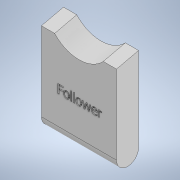
# Autodesk Inventor part: Follower
Saved by Autodesk Inventor 2021 (Build 250183000, 183)
## iProperties
Created: 2021-04-12
Part Number: Follower
Material: Generic
Document SubType Name: Modeling
Designer: Nabeel Azafer
Density: 1 g/cm^3
Appearance: Default
Author: Nabeel Azafer
Autodesk Inventor part; units mm, degrees
note: some values were not read from the file. Chosen so that the rebuilt part matches the saved one: direction of "Emboss1".
ref_plane "YZ Plane" through (0, 0, 0) normal (1, 0, 0) x (0, 1, 0)
ref_plane "XZ Plane" through (0, 0, 0) normal (0, 1, 0) x (-1, 0, 0)
sketch "Sketch1" plane through (0, 0, 0) normal (0, 0, 1) x (1, 0, 0)
  line L0 (0, 0) -> (17, 0)
  line L1 (17, 0) -> (17, 21.5)
  line L2 (17, 21.5) -> (0, 21.5)
  line L3 (0, 21.5) -> (0, 0)
  dimension "d0" = 17
  dimension "d1" = 21.5
  constraints: 8 end point, 2 parallel, 1 horizontal, 1 perpendicular
  measures "d0" distance of L0.start L0.end
  measures "d1" distance of L2.end L0.start
extrude "Extrusion1" add sketch "Sketch1" along normal blind 5
fillet "Fillet2" radius 2.5 2 edges at (8.5, 0, 5) (8.5, 0, 0)
ref_plane "Work Plane1" through (8.5, 21.5, 0) normal (-1, 0, 0) x (0, 0, 1)
sketch "Sketch5" plane through (8.5, 21.5, 0) normal (-1, 0, 0) x (0, 0, 1)
  line L0 (0, 0) -> (5, -1.1543)
  line L1 (5, -19) -> (5, 0) projected
  line L2 (0, 0) -> (5.1315, 0) construction
  point P0 (0, -21.5)
  dimension "d22" = 13
  constraints: 4 end point, 1 equal length, 1 horizontal, 1 point on line
  measures "d22" angle of L0 L2
sketch "Sketch6" plane through (0, 0, 0) normal (0, 0, -1) x (-1, 0, 0)
  line L0 (-14, 21.5) -> (-14, 24.5)
  line L1 (-14, 24.5) -> (-3, 24.5)
  line L2 (-3, 24.5) -> (-3, 21.5)
  line L3 (-17, 21.5) -> (0, 21.5) projected
  arc A0 (-14, 21.5) -> (-3, 21.5) centre (-8.5, 26.599) ccw
  point P0 (0, 0)
  dimension "d27" = 3
  dimension "d31" = 3
  dimension "d32" = 3
  dimension "d33" = 3
  dimension "d34" = 7.5
  constraints: 6 end point, 2 perpendicular, 2 point on circle, 1 centre point, 1 vertical
  measures "d27" distance of L0.start L0.end
  measures "d31" distance from line of L3.end L2
  measures "d32" distance between parallel lines of L3 L1
  measures "d33" distance of L1.end L2.end
  measures "d34" radius of A0
sweep "Sweep1" cut profiles "Sketch6" path "Sketch5" path curves L0
sketch "Sketch8" plane through (17, 21.5, 5) normal (1, 0, 0) x (0, 0, -1)
  line L0 (5, 0) -> (0, 0) projected
  line L1 (5, 0) -> (0, -1.1543) projected
  line L2 (5, 0) -> (0, -1.1543)
  line L3 (0, -19) -> (0, 0) projected
  line L4 (0, -1.1543) -> (0, 0)
  line L5 (0, 0) -> (5, 0)
  point P0 (5, -21.5)
  constraints: 6 end point, 2 collinear, 1 perpendicular
extrude "Extrusion6" cut sketch "Sketch8" against normal blind 17
sketch "Sketch9" plane through (0, 0, 5) normal (0, 0, 1) x (1, 0, 0)
  line L0 (3.5412, 10.9902) -> (19.7264, 10.9902) construction
  line L1 (19.7264, 10.9902) -> (19.7264, 4.3416) construction
  line L2 (19.7264, 4.3416) -> (3.5412, 4.3416) construction
  line L3 (3.5412, 4.3416) -> (3.5412, 10.9902) construction
  line L4 (4.9399, 10.6645) -> (4.0096, 10.6645)
  line L5 (4.0096, 10.6645) -> (4.0096, 10.1004)
  line L6 (4.0096, 10.1004) -> (4.901, 10.1004)
  line L7 (4.901, 10.1004) -> (4.901, 9.8638)
  line L8 (4.901, 9.8638) -> (4.0096, 9.8638)
  line L9 (4.0096, 9.8638) -> (4.0096, 8.9011)
  line L10 (4.0096, 8.9011) -> (3.7438, 8.9011)
  line L11 (3.7438, 8.9011) -> (3.7438, 10.9011)
  line L12 (3.7438, 10.9011) -> (4.9399, 10.9011)
  line L13 (4.9399, 10.9011) -> (4.9399, 10.6645)
  spline S0 degree 2 poles (6.3921, 9.6515) (6.3921, 9.2722) (6.0275, 8.859) (5.7228, 8.859) knots 0 0 0 1 2 2 2
  spline S1 degree 2 poles (5.7228, 8.859) (5.41, 8.859) (5.0518, 9.2852) (5.0518, 9.6515) knots 0 0 0 1 2 2 2
  spline S2 degree 2 poles (5.0518, 9.6515) (5.0518, 10.0275) (5.4213, 10.444) (5.7228, 10.444) knots 0 0 0 1 2 2 2
  spline S3 degree 2 poles (5.7228, 10.444) (6.0275, 10.444) (6.3921, 10.0291) (6.3921, 9.6515) knots 0 0 0 1 2 2 2
  spline S4 degree 2 poles (6.1312, 9.6515) (6.1312, 9.9432) (5.9189, 10.2269) (5.7228, 10.2269) knots 0 0 0 1 2 2 2
  spline S5 degree 2 poles (5.7228, 10.2269) (5.5266, 10.2269) (5.3127, 9.9432) (5.3127, 9.6515) knots 0 0 0 1 2 2 2
  spline S6 degree 2 poles (5.3127, 9.6515) (5.3127, 9.3679) (5.5266, 9.0761) (5.7228, 9.0761) knots 0 0 0 1 2 2 2
  spline S7 degree 2 poles (5.7228, 9.0761) (5.9172, 9.0761) (6.1312, 9.363) (6.1312, 9.6515) knots 0 0 0 1 2 2 2
  line L14 (6.9091, 8.9011) -> (6.6563, 8.9011)
  line L15 (6.6563, 8.9011) -> (6.6563, 10.9902)
  line L16 (6.6563, 10.9902) -> (6.9091, 10.9902)
  line L17 (6.9091, 10.9902) -> (6.9091, 8.9011)
  line L18 (7.538, 8.9011) -> (7.2852, 8.9011)
  line L19 (7.2852, 8.9011) -> (7.2852, 10.9902)
  line L20 (7.2852, 10.9902) -> (7.538, 10.9902)
  line L21 (7.538, 10.9902) -> (7.538, 8.9011)
  spline S8 degree 2 poles (9.1425, 9.6515) (9.1425, 9.2722) (8.7779, 8.859) (8.4732, 8.859) knots 0 0 0 1 2 2 2
  spline S9 degree 2 poles (8.4732, 8.859) (8.1604, 8.859) (7.8022, 9.2852) (7.8022, 9.6515) knots 0 0 0 1 2 2 2
  spline S10 degree 2 poles (7.8022, 9.6515) (7.8022, 10.0275) (8.1717, 10.444) (8.4732, 10.444) knots 0 0 0 1 2 2 2
  spline S11 degree 2 poles (8.4732, 10.444) (8.7779, 10.444) (9.1425, 10.0291) (9.1425, 9.6515) knots 0 0 0 1 2 2 2
  spline S12 degree 2 poles (8.8816, 9.6515) (8.8816, 9.9432) (8.6693, 10.2269) (8.4732, 10.2269) knots 0 0 0 1 2 2 2
  spline S13 degree 2 poles (8.4732, 10.2269) (8.2771, 10.2269) (8.0631, 9.9432) (8.0631, 9.6515) knots 0 0 0 1 2 2 2
  spline S14 degree 2 poles (8.0631, 9.6515) (8.0631, 9.3679) (8.2771, 9.0761) (8.4732, 9.0761) knots 0 0 0 1 2 2 2
  spline S15 degree 2 poles (8.4732, 9.0761) (8.6677, 9.0761) (8.8816, 9.363) (8.8816, 9.6515) knots 0 0 0 1 2 2 2
  line L22 (11.2203, 10.4019) -> (10.8395, 8.9011)
  line L23 (10.8395, 8.9011) -> (10.6061, 8.9011)
  line L24 (10.6061, 8.9011) -> (10.2398, 10.0583)
  line L25 (10.2398, 10.0583) -> (9.8751, 8.9011)
  line L26 (9.8751, 8.9011) -> (9.6433, 8.9011)
  line L27 (9.6433, 8.9011) -> (9.2592, 10.4019)
  line L28 (9.2592, 10.4019) -> (9.5218, 10.4019)
  line L29 (9.5218, 10.4019) -> (9.7876, 9.2398)
  line L30 (9.7876, 9.2398) -> (10.1425, 10.4019)
  line L31 (10.1425, 10.4019) -> (10.3516, 10.4019)
  line L32 (10.3516, 10.4019) -> (10.7163, 9.2398)
  line L33 (10.7163, 9.2398) -> (10.9659, 10.4019)
  line L34 (10.9659, 10.4019) -> (11.2203, 10.4019)
  spline S16 degree 2 poles (12.0939, 8.8671) (11.7341, 8.8671) (11.3386, 9.2706) (11.3386, 9.6434) knots 0 0 0 1 2 2 2
  spline S17 degree 2 poles (11.3386, 9.6434) (11.3386, 10.0097) (11.7228, 10.444) (12.0323, 10.444) knots 0 0 0 1 2 2 2
  spline S18 degree 2 poles (12.0323, 10.444) (12.1717, 10.444) (12.3873, 10.363) (12.4667, 10.2771) knots 0 0 0 1 2 2 2
  spline S19 degree 2 poles (12.4667, 10.2771) (12.5477, 10.1912) (12.6336, 9.9432) (12.6336, 9.7633) knots 0 0 0 1 2 2 2
  line L35 (12.6336, 9.7633) -> (12.6336, 9.6256)
  line L36 (12.6336, 9.6256) -> (11.5947, 9.6256)
  spline S20 degree 2 poles (11.5947, 9.6256) (11.5947, 9.3646) (11.8573, 9.0875) (12.0907, 9.0875) knots 0 0 0 1 2 2 2
  spline S21 degree 2 poles (12.0907, 9.0875) (12.1733, 9.0875) (12.3338, 9.1248) (12.3986, 9.1539) knots 0 0 0 1 2 2 2
  spline S22 degree 2 poles (12.3986, 9.1539) (12.4667, 9.1863) (12.5607, 9.2431) (12.5915, 9.269) knots 0 0 0 1 2 2 2
  line L37 (12.5915, 9.269) -> (12.6061, 9.269)
  line L38 (12.6061, 9.269) -> (12.6061, 8.9935)
  spline S23 degree 2 poles (12.6061, 8.9935) (12.5623, 8.9756) (12.4294, 8.9238) (12.3775, 8.9092) knots 0 0 0 1 2 2 2
  spline S24 degree 2 poles (12.3775, 8.9092) (12.3046, 8.8881) (12.1847, 8.8671) (12.0939, 8.8671) knots 0 0 0 1 2 2 2
  spline S25 degree 2 poles (12.3873, 9.8184) (12.384, 9.9205) (12.3419, 10.0696) (12.3014, 10.1199) knots 0 0 0 1 2 2 2
  spline S26 degree 2 poles (12.3014, 10.1199) (12.2576, 10.1766) (12.1198, 10.2366) (12.0177, 10.2366) knots 0 0 0 1 2 2 2
  spline S27 degree 2 poles (12.0177, 10.2366) (11.9172, 10.2366) (11.7762, 10.1766) (11.7179, 10.1183) knots 0 0 0 1 2 2 2
  spline S28 degree 2 poles (11.7179, 10.1183) (11.6612, 10.0583) (11.6028, 9.9141) (11.5947, 9.8184) knots 0 0 0 1 2 2 2
  line L39 (11.5947, 9.8184) -> (12.3873, 9.8184)
  line L40 (13.6855, 10.1312) -> (13.6725, 10.1312)
  spline S29 degree 2 poles (13.6725, 10.1312) (13.6433, 10.1393) (13.5801, 10.1426) (13.5364, 10.1426) knots 0 0 0 1 2 2 2
  spline S30 degree 2 poles (13.5364, 10.1426) (13.4343, 10.1426) (13.2333, 10.0534) (13.1425, 9.9659) knots 0 0 0 1 2 2 2
  line L41 (13.1425, 9.9659) -> (13.1425, 8.9011)
  line L42 (13.1425, 8.9011) -> (12.8897, 8.9011)
  line L43 (12.8897, 8.9011) -> (12.8897, 10.4019)
  line L44 (12.8897, 10.4019) -> (13.1425, 10.4019)
  line L45 (13.1425, 10.4019) -> (13.1425, 10.1782)
  spline S31 degree 2 poles (13.1425, 10.1782) (13.2803, 10.3014) (13.4861, 10.4019) (13.5834, 10.4019) knots 0 0 0 1 2 2 2
  spline S32 degree 2 poles (13.5834, 10.4019) (13.6223, 10.4019) (13.6612, 10.3987) (13.6855, 10.3938) knots 0 0 0 1 2 2 2
  line L46 (13.6855, 10.3938) -> (13.6855, 10.1312)
  point P0 (0, 0)
  constraints: 2 other
emboss "Emboss1" sketch "Sketch9" operation cut depth 1 direction (0, 0, -1)
body "Solid1"
